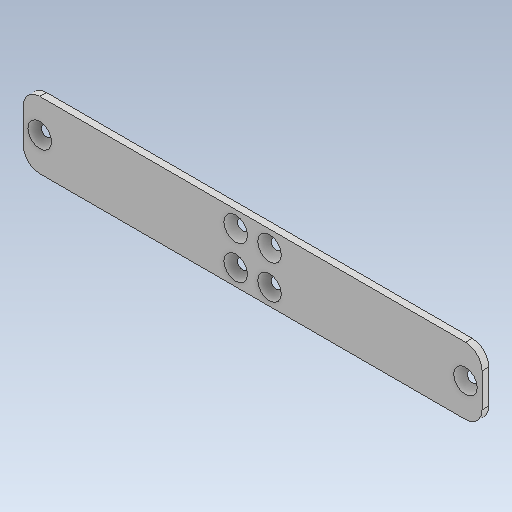
# Autodesk Inventor part: РеброСкрепления
Saved by Autodesk Inventor 2020 (Build 240168000, 168)
## iProperties
Created: 2021-02-25
Part Number: РеброСкрепления
Material: Типовые
Document SubType Name: Modeling
Designer: I_Love_U_Bogdan
Density: 1 g/cm^3
Appearance: По умолчанию
Author: I_Love_U_Bogdan
Autodesk Inventor part; units mm, degrees
ref_plane "YZ Plane" through (0, 0, 0) normal (1, 0, 0) x (0, 1, 0)
ref_plane "XZ Plane" through (0, 0, 0) normal (0, 1, 0) x (-1, 0, 0)
ref_plane "XY Plane" through (0, 0, 0) normal (0, 0, 1) x (1, 0, 0)
sketch "Эскиз1" plane through (0, 0, 0) normal (0, 0, 1) x (1, 0, 0)
  circle A0 centre (37.4694, -15.6747) radius 1.5 projected
  circle A1 centre (-20.5306, -10.6747) radius 1.5 projected
  circle A2 centre (-20.5306, -20.6747) radius 1.5 projected
  arc A3 (37.4694, -25.6747) -> (42.4694, -20.6747) centre (37.4694, -20.6747) ccw projected
  line L0 (42.4694, -10.6747) -> (42.4694, -20.6747) projected
  arc A4 (42.4694, -10.6747) -> (37.4694, -5.6747) centre (37.4694, -10.6747) ccw projected
  line L1 (-25.5306, -5.6747) -> (37.4694, -5.6747) projected
  line L2 (-25.5306, -25.6747) -> (-25.5306, -5.6747) projected
  line L3 (37.4694, -25.6747) -> (-25.5306, -25.6747) projected
  arc A5 (42.3694, -10.6747) -> (37.4694, -5.7747) centre (37.4694, -10.6747) ccw
  line L4 (42.3694, -10.6747) -> (42.3694, -20.6747)
  arc A6 (37.4694, -25.5747) -> (42.3694, -20.6747) centre (37.4694, -20.6747) ccw
  line L5 (37.4694, -25.5747) -> (-25.5306, -25.5747)
  line L6 (-25.5306, -5.7747) -> (37.4694, -5.7747)
  point P0 (0, 0)
  dimension "d0" = 0.1
  constraints: 6 end point, 4 point on circle, 2 centre point, 2 point on line, 2 other
  measures "d0" distance between parallel lines of L1 L6
extrude "Выдавливание1" add sketch "Эскиз1" along normal blind 2 contours L2 L6 A5 L4 A6 L5
chamfer "Фаска1" distance 2 angle 45 3 edges at (35.9694, -15.6747, 2) (-22.0306, -20.6747, 2) (-22.0306, -10.6747, 2)
mirror "Зеркальное отражение1" about plane through (-25.5306, -5.7747, 0) normal (-1, 0, 0)
